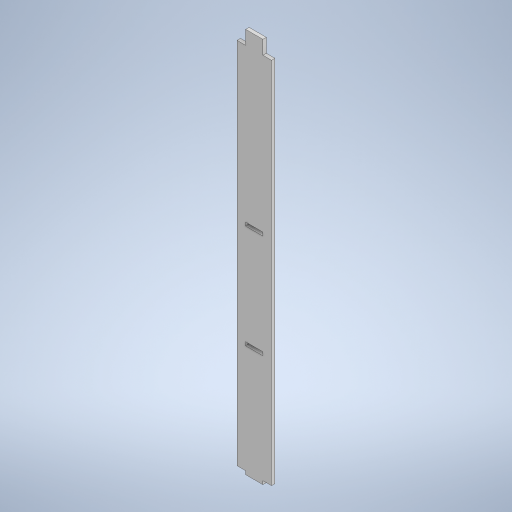
# Autodesk Inventor part: back_down_hold
Saved by Autodesk Inventor 2024 (Build 280153000, 153)
## iProperties
Created: 2024-03-23
Part Number: back_down_hold
Material: Generic
Document SubType Name: Modeling
Designer: op04o
Density: 1 g/cm^3
Appearance: Default
Author: op04o
Autodesk Inventor part; units mm, degrees
ref_plane "YZ Plane" through (0, 0, 0) normal (1, 0, 0) x (0, 1, 0)
ref_plane "XZ Plane" through (0, 0, 0) normal (0, 1, 0) x (-1, 0, 0)
ref_plane "XY Plane" through (0, 0, 0) normal (0, 0, 1) x (1, 0, 0)
sketch "Sketch1" plane through (0, 0, 0) normal (0, 0, 1) x (1, 0, 0)
  line L0 (0, 0) -> (15, 0)
  line L1 (15, 0) -> (15, 12)
  line L2 (15, 12) -> (0, 12)
  line L3 (0, 12) -> (0, 0)
  line L4 (-7.5, 0) -> (22.5, 0)
  line L5 (22.5, 0) -> (22.5, -320)
  line L6 (-7.5, -320) -> (-7.5, 0)
  line L7 (0, -133) -> (15, -133)
  line L8 (15, -133) -> (15, -136)
  line L9 (15, -136) -> (0, -136)
  line L10 (0, -136) -> (0, -133)
  line L11 (15, -320) -> (15, -323)
  line L12 (15, -323) -> (0, -323)
  line L13 (0, -323) -> (0, -320)
  line L14 (22.5, -320) -> (15, -320)
  line L15 (0, -320) -> (-7.5, -320)
  line L16 (0, -223) -> (15, -223)
  line L17 (15, -223) -> (15, -226)
  line L18 (15, -226) -> (0, -226)
  line L19 (0, -226) -> (0, -223)
  point P0 (7.5, 12)
  point P1 (7.5, -320)
  point P2 (7.5, -133)
  point P3 (7.5, 0)
  point P4 (7.5, -323)
  point P5 (7.5, -223)
  dimension "d0" = 15
  dimension "d1" = 12
  dimension "d3" = 30
  dimension "d6" = 3
  dimension "d8" = 15
  dimension "d9" = 15
  dimension "d11" = 7.5
  dimension "d13" = 22.5
  dimension "d15" = 145
  dimension "d16" = 3
  dimension "d17" = 320
  dimension "d18" = 7.5
  dimension "d21" = 22.5
  dimension "d23" = 15
  dimension "d24" = 3
  dimension "d26" = 90
  constraints: 40 end point, 12 parallel, 5 midpoint, 4 horizontal, 4 perpendicular, 4 vertical alignment, 2 equal length, 1 horizontal alignment, 1 point on line
  measures "d0" distance of L2.end L1.end
  measures "d1" distance of L1.end L0.end
  measures "d3" distance of L5.end L6.start
  measures "d6" distance of L7.end L8.end
  measures "d8" distance of L8.end L9.end
  measures "d9" distance of L11.end L12.end
  measures "d11" distance from line of point (15, 0) L5
  measures "d13" distance from line of point (0, 0) L5
  measures "d15" distance of L1.end L7.end
  measures "d16" vertical distance of L5.end L11.end
  measures "d17" distance between parallel lines of L4 L14
  measures "d18" distance from line of point (15, 0) L5
  measures "d21" distance from line of point (0, 0) L5
  measures "d23" distance of L16.start L16.end
  measures "d24" distance of L18.end L16.start
  measures "d26" distance of L16.end L7.end
extrude "Extrusion1" add sketch "Sketch1" along normal blind 3
body "Solid1"
